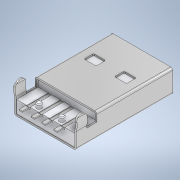
# Autodesk Inventor part: USB
Saved by Autodesk Inventor 2020 (Build 240168000, 168)
## iProperties
Created: 2022-06-10
Part Number: USB
Material: Типовые
Document SubType Name: Modeling
Designer: NoName
Density: 1 g/cm^3
Appearance: По умолчанию
Author: NoName
Autodesk Inventor part; units mm, degrees
ref_plane "YZ Plane" through (0, 0, 0) normal (1, 0, 0) x (0, 1, 0)
ref_plane "XZ Plane" through (0, 0, 0) normal (0, 1, 0) x (-1, 0, 0)
ref_plane "XY Plane" through (0, 0, 0) normal (0, 0, 1) x (1, 0, 0)
sketch "Эскиз1" plane through (0, 0, 0) normal (0, 0, 1) x (1, 0, 0)
  line L0 (-6, -2.25) -> (6, -2.25)
  line L1 (6, -2.25) -> (6, 2.25)
  line L2 (6, 2.25) -> (-6, 2.25)
  line L3 (-6, 2.25) -> (-6, -2.25)
  line L4 (-6, -2.25) -> (6, 2.25) construction
  line L5 (6, -2.25) -> (-6, 2.25) construction
  point P0 (0, 0)
  dimension "d0" = 12
  dimension "d1" = 4.5
  constraints: 12 end point, 2 midpoint, 2 parallel, 1 horizontal, 1 perpendicular
  measures "d0" distance between parallel lines of L1 L3
  measures "d1" distance between parallel lines of L0 L2
extrude "Выдавливание1" add sketch "Эскиз1" along normal blind 18.75
fillet "Сопряжение1" radius 0.4 4 edges at (6, 2.25, 9.375) (6, -2.25, 9.375) (-6, 2.25, 9.375) (-6, -2.25, 9.375)
shell "Оболочка1" thickness 0.3 removed faces 2 at (1.8667, -0.75, 18.75) at (1.8667, -0.75, 0)
sketch "Эскиз7" plane through (-5.6, -2.25, 0) normal (0, -1, 0) x (1, 0, 0)
  line L0 (1.675, 5.25) -> (3.6, 5.25)
  line L1 (3.8, 5.45) -> (3.8, 6.9)
  line L2 (3.6, 7.1) -> (1.675, 7.1)
  line L3 (1.475, 6.9) -> (1.475, 5.45)
  line L4 (7.6, 5.25) -> (9.525, 5.25)
  line L5 (9.725, 5.45) -> (9.725, 6.9)
  line L6 (9.525, 7.1) -> (7.6, 7.1)
  line L7 (7.4, 6.9) -> (7.4, 5.45)
  line L8 (5.6, 0) -> (5.6, 18.75)
  line L9 (0, 18.75) -> (11.2, 18.75) projected
  line L10 (0, 0) -> (11.2, 0) projected
  arc A0 (1.675, 7.1) -> (1.475, 6.9) centre (1.675, 6.9) ccw
  arc A1 (3.8, 6.9) -> (3.6, 7.1) centre (3.6, 6.9) ccw
  arc A2 (3.6, 5.25) -> (3.8, 5.45) centre (3.6, 5.45) ccw
  arc A3 (1.475, 5.45) -> (1.675, 5.25) centre (1.675, 5.45) ccw
  arc A4 (7.4, 5.45) -> (7.6, 5.25) centre (7.6, 5.45) ccw
  arc A5 (7.6, 7.1) -> (7.4, 6.9) centre (7.6, 6.9) ccw
  arc A6 (9.725, 6.9) -> (9.525, 7.1) centre (9.525, 6.9) ccw
  arc A7 (9.525, 5.25) -> (9.725, 5.45) centre (9.525, 5.45) ccw
  point P0 (1.475, 5.25)
  point P1 (3.8, 7.1)
  point P2 (3.8, 5.25)
  point P3 (1.475, 7.1)
  point P4 (7.4, 5.25)
  point P5 (9.725, 7.1)
  point P6 (9.725, 5.25)
  point P7 (7.4, 7.1)
  dimension "d32" = 3.6
  dimension "d33" = 8.25
  dimension "d34" = 1.85
  dimension "d35" = 5.25
  dimension "d38" = 0.2
  constraints: 18 end point, 16 point on circle, 16 point on line, 16 tangent, 8 centre point, 7 equal radius, 4 parallel, 2 horizontal, 2 perpendicular, 1 midpoint, 4 other
  measures "d32" distance between parallel lines of L7 L1
  measures "d33" distance between parallel lines of L5 L3
  measures "d34" distance between parallel lines of L0 L2
  measures "d35" distance between parallel lines of L10 L0
  measures "d38" radius of A0
extrude "Выдавливание6" cut sketch "Эскиз7" against normal through all
sketch "Эскиз5" plane through (0, 0, 0) normal (1, 0, 0) x (0, 1, 0)
  line L0 (2.25, 0) -> (1.85, 0) projected
  line L1 (1.95, 0.1) -> (-0.05, 0.1)
  line L2 (-0.05, 0.1) -> (-0.05, 8.6)
  line L3 (-0.05, 8.6) -> (1.95, 8.6)
  line L4 (1.95, 8.6) -> (1.95, 0)
  line L5 (-1.95, 0) -> (-1.95, 18.75) projected
  line L6 (1.95, 8.6) -> (-1.95, 8.6)
  line L7 (-1.95, 8.6) -> (-1.95, 14.45)
  line L8 (-1.95, 14.45) -> (1.95, 14.45)
  line L9 (1.95, 14.45) -> (1.95, 8.6)
  line L10 (-1.95, 14.45) -> (0.45, 14.45)
  line L11 (0.45, 14.45) -> (0.45, 18.65)
  line L12 (0.45, 18.65) -> (-1.95, 18.65)
  line L13 (-1.95, 18.65) -> (-1.95, 14.45)
  line L14 (1.95, 18.75) -> (1.95, 0) projected
  line L15 (1.85, 0) -> (-1.85, 0) projected
  line L16 (-1.85, 18.75) -> (1.85, 18.75) projected
  line L17 (-2.25, 0) -> (-2.25, 18.75) projected
  point P0 (0, 0)
  dimension "d20" = 2
  dimension "d21" = 0.1
  dimension "d22" = 0.1
  dimension "d23" = 8.6
  dimension "d24" = 4.3
  dimension "d25" = 2.7
  constraints: 24 end point, 6 parallel, 4 point on line, 3 horizontal, 3 perpendicular
  measures "d20" distance between parallel lines of L4 L2
  measures "d21" distance between parallel lines of L15 L1
  measures "d22" distance between parallel lines of L16 L12
  measures "d23" distance between parallel lines of L15 L6
  measures "d24" distance between parallel lines of L16 L8
  measures "d25" distance between parallel lines of L17 L11
extrude "Выдавливание4" add sketch "Эскиз5" along normal mid plane 11.5
sketch "Эскиз6" plane through (-6, -1.85, 0) normal (-1, 0, 0) x (0, 0, 1)
  line L0 (14.75, 2.4) -> (18.75, 2.4)
  line L1 (18.75, 2.4) -> (18.75, 4.1)
  line L2 (18.75, 4.1) -> (14.75, 4.1)
  line L3 (14.75, 4.1) -> (14.75, 2.4)
  line L4 (0, -0.4) -> (18.75, -0.4) projected
  point P0 (0, 1.85)
  dimension "d28" = 2.8
  dimension "d29" = 4
  constraints: 8 end point, 2 parallel, 1 coincident, 1 horizontal, 1 perpendicular
  measures "d28" distance between parallel lines of L4 L0
  measures "d29" distance between parallel lines of L1 L3
extrude "Выдавливание5" cut sketch "Эскиз6" against normal through all
sketch "Эскиз8" plane through (-5.7, 0.45, 18.65) normal (0, 1, 0) x (1, 0, 0)
  circle A0 centre (7.9, 0.9) radius 0.5
  circle A1 centre (3.5, 0.9) radius 0.5
  line L0 (11.3, 3.9) -> (0.1, 3.9) projected
  line L1 (5.7, 3.9) -> (5.7, -0.1)
  line L2 (11.3, -0.1) -> (0.1, -0.1) projected
  point P0 (5.7, 18.65)
  dimension "d39" = 1
  dimension "d40" = 4.4
  dimension "d41" = 1
  constraints: 2 centre point, 2 end point, 2 midpoint, 1 equal radius, 1 other
  measures "d39" diameter of A0
  measures "d40" distance of A1.centre A0.centre
  measures "d41" distance from line of L2 A1.centre
extrude "Выдавливание7" add sketch "Эскиз8" along normal blind 0.8
chamfer "Фаска2" distance 0.15 angle 45 2 edges at (1.7, 1.25, 17.75) (-2.7, 1.25, 17.75)
sketch "Эскиз9" plane through (-5.7, 0.45, 18.65) normal (0, 1, 0) x (1, 0, 0)
  line L0 (11.4, 4.2) -> (0, 4.2) projected
  line L1 (0, 0) -> (11.4, 0) construction
  line L2 (9.4, 4.2) -> (8.75, 4.2)
  line L3 (8.75, 4.2) -> (8.75, 0)
  line L4 (8.75, 0) -> (9.4, 0)
  line L5 (9.4, 0) -> (9.4, 4.2)
  line L6 (7.05, 0) -> (6.4, 0)
  line L7 (6.4, 0) -> (6.4, 4.2)
  line L8 (6.4, 4.2) -> (7.05, 4.2)
  line L9 (7.05, 4.2) -> (7.05, 0)
  line L10 (11.7, 3.9) -> (11.7, -0.1) projected
  line L11 (5.7, 4.2) -> (5.7, 0)
  line L12 (2, 4.2) -> (2.65, 4.2)
  line L13 (2.65, 4.2) -> (2.65, 0)
  line L14 (2.65, 0) -> (2, 0)
  line L15 (2, 0) -> (2, 4.2)
  line L16 (4.35, 0) -> (5, 0)
  line L17 (5, 0) -> (5, 4.2)
  line L18 (5, 4.2) -> (4.35, 4.2)
  line L19 (4.35, 4.2) -> (4.35, 0)
  point P0 (5.7, 18.65)
  dimension "d47" = 0.65
  dimension "d48" = 0.65
  dimension "d49" = 4.65
  dimension "d50" = 2.3
  constraints: 34 end point, 8 symmetric about line, 6 point on line, 4 parallel, 2 horizontal, 2 midpoint, 2 perpendicular
  measures "d47" distance between parallel lines of L7 L9
  measures "d48" distance between parallel lines of L5 L3
  measures "d49" distance between parallel lines of L10 L9
  measures "d50" distance between parallel lines of L10 L5
extrude "Выдавливание8" cut sketch "Эскиз9" against normal blind 0.1
sketch "Эскиз10" plane through (3.05, 0.45, 18.65) normal (1, 0, 0) x (0, 0, -1)
  line L0 (0, 0) -> (4.2, 0) projected
  line L1 (0, -0.1) -> (4.2, -0.1) projected
  line L2 (4.2, 0) -> (4.2, -0.1) projected
  line L3 (0, -0.1) -> (-0.1414, 0.0414)
  line L4 (-0.2828, 0.1) -> (-1.5, 0.1)
  line L5 (0, -2.3) -> (0, 0) projected
  line L6 (-1.5, 0.1) -> (-1.5, -0.1)
  line L7 (-1.5, -0.1) -> (-0.3657, -0.1)
  line L8 (-0.2243, -0.1586) -> (0, -0.3828)
  line L9 (-0.1, -2.3) -> (-0.1, 0.1) projected
  arc A0 (-0.1414, 0.0414) -> (-0.2828, 0.1) centre (-0.2828, -0.1) ccw
  arc A1 (-0.2243, -0.1586) -> (-0.3657, -0.1) centre (-0.3657, -0.3) ccw
  line L10 (0, -0.1) -> (0, 0) projected
  point P0 (18.65, -0.45)
  point P1 (-0.2828, -0.1)
  dimension "d54" = 0.2
  dimension "d55" = 0.2
  dimension "d56" = 1.4
  dimension "d57" = 0.2
  constraints: 10 end point, 4 point on circle, 4 tangent, 3 perpendicular, 3 point on line, 2 centre point, 1 equal radius, 1 horizontal alignment, 1 parallel
  measures "d54" distance between parallel lines of L4 L7
  measures "d55" distance between parallel lines of L3 L8
  measures "d56" distance between parallel lines of L9 L6
  measures "d57" radius of A0
extrude "Выдавливание9" add sketch "Эскиз10" along normal up to surface (0.65 mm away) contours L5 L8 L9 L3 | L9 L8 A1 L7 L6 L4 A0 L3
chamfer "Фаска3" distance 0.6 angle 45 1 edges at (0, -0.05, 0.1)
sketch "Эскиз11" plane through (-5.7, -0.05, 8.6) normal (0, -1, 0) x (1, 0, 0)
  line L0 (11.4, -7.9) -> (0, -7.9) projected
  line L1 (11.4, 0) -> (11.4, -7.9) projected
  line L2 (0, 0) -> (11.4, 0) projected
  line L3 (0, -7.9) -> (0, 0) projected
  line L4 (8.75, 10.05) -> (8.75, 5.85) projected
  line L5 (9.4, 5.85) -> (9.4, 10.05) projected
  line L6 (8.75, 5.85) -> (9.4, 5.85) projected
  line L7 (7.05, 5.85) -> (7.05, 10.05) projected
  line L8 (6.4, 5.85) -> (7.05, 5.85) projected
  line L9 (6.4, 10.05) -> (6.4, 5.85) projected
  line L10 (5, 5.85) -> (5, 10.05) projected
  line L11 (4.35, 5.85) -> (5, 5.85) projected
  line L12 (4.35, 10.05) -> (4.35, 5.85) projected
  line L13 (2.65, 5.85) -> (2.65, 10.05) projected
  line L14 (2, 5.85) -> (2.65, 5.85) projected
  line L15 (2, 10.05) -> (2, 5.85) projected
  line L16 (0.1, 0) -> (11.3, 0) projected
  line L17 (9.675, 0) -> (8.475, 0)
  line L18 (8.475, 0) -> (8.475, -7.6)
  line L19 (8.475, -7.6) -> (9.675, -7.6)
  line L20 (9.675, -7.6) -> (9.675, 0)
  line L21 (0.1, -8.6) -> (11.3, -8.6) projected
  line L22 (7.325, 0) -> (6.125, 0)
  line L23 (6.125, 0) -> (6.125, -6.1)
  line L24 (6.125, -6.1) -> (7.325, -6.1)
  line L25 (7.325, -6.1) -> (7.325, 0)
  line L26 (5.7, -8.6) -> (5.7, 0)
  line L27 (1.725, 0) -> (2.925, 0)
  line L28 (2.925, 0) -> (2.925, -7.6)
  line L29 (2.925, -7.6) -> (1.725, -7.6)
  line L30 (1.725, -7.6) -> (1.725, 0)
  line L31 (4.075, 0) -> (5.275, 0)
  line L32 (5.275, 0) -> (5.275, -6.1)
  line L33 (5.275, -6.1) -> (4.075, -6.1)
  line L34 (4.075, -6.1) -> (4.075, 0)
  line L35 (2.65, 10.05) -> (2, 10.05) projected
  line L36 (5, 10.05) -> (4.35, 10.05) projected
  line L37 (7.05, 10.05) -> (6.4, 10.05) projected
  line L38 (9.4, 10.05) -> (8.75, 10.05) projected
  point P0 (9.075, 0)
  point P1 (9.075, 5.85)
  point P2 (6.725, 0)
  point P3 (6.725, 5.85)
  point P4 (2.325, 0)
  point P5 (4.675, 0)
  point P6 (9.675, 0)
  point P7 (8.475, 0)
  point P8 (2.925, 0)
  point P9 (1.725, 0)
  dimension "d63" = 1.2
  dimension "d64" = 1
  dimension "d65" = 2.5
  constraints: 34 end point, 10 symmetric about line, 5 midpoint, 5 parallel, 2 horizontal, 2 perpendicular, 2 point on line, 2 vertical alignment
  measures "d63" distance between parallel lines of L18 L20
  measures "d64" distance between parallel lines of L21 L19
  measures "d65" distance between parallel lines of L21 L24
extrude "Выдавливание10" cut sketch "Эскиз11" against normal blind 0.1 contours L32 L33 L34 L2 | L2 L25 L24 L23 | L20 L19 L18 L2 | L2 L28 L29 L30
pattern_linear "Прямоуг.массив1" count 2 spacing 2.35 along (-1, 0, 0) of "Выдавливание9"
mirror "Зеркальное отражение1" about plane through (0, 0, 0) normal (1, 0, 0) of "Выдавливание9", "Прямоуг.массив1"
sketch "Эскиз12" plane through (0, 0, 18.75) normal (0, 0, 1) x (1, 0, 0)
  line L0 (6, 1.85) -> (6, 0.55) projected
  line L1 (6, 0.55) -> (5.7, 0.55)
  line L2 (5.7, 0.55) -> (5.7, 3.45) construction
  line L3 (5.7, 3.45) -> (6, 3.45)
  line L4 (6, 3.45) -> (6, 0.55) construction
  line L5 (-5.6, -2.25) -> (5.6, -2.25) projected
  arc A0 (6, 0.944) -> (6, 3.056) centre (3.192, 2) ccw
  line L6 (5.7, 0.55) -> (5.7, 1.85) projected
  arc A1 (5.7, 1) -> (5.7, 3) centre (3.192, 2) ccw
  line L7 (5.7, 3) -> (5.7, 3.45)
  line L8 (6, 3.45) -> (6, 3.056)
  line L9 (6, 0.944) -> (6, 0.55)
  line L10 (6, -1.85) -> (6, 1.85) projected
  line L11 (5.7, 1) -> (5.7, 0.55)
  line L12 (5.7, -1.85) -> (5.7, 1.85) projected
  point P0 (0, 0)
  point P1 (6, 0.944)
  dimension "d84" = 5.7
  dimension "d85" = 0.3
  dimension "d86" = 3
  dimension "d87" = 2
  dimension "d88" = 4.25
  constraints: 16 end point, 5 point on line, 4 point on circle, 3 collinear, 2 centre point, 2 parallel, 1 coincident, 1 horizontal, 1 perpendicular, 1 vertical
  measures "d84" distance between parallel lines of L3 L5
  measures "d85" radial gap between concentric circles of A0 A1
  measures "d86" radius of A0
  measures "d87" distance of L11.start L7.start
  measures "d88" distance from line of L5 A0.centre
extrude "Выдавливание11" add sketch "Эскиз12" against normal blind 2
sketch "Эскиз14" plane through (5.7, 3, 18.75) normal (-1, 0, 0) x (0, 0, 1)
  line L0 (-2, -2) -> (-2, 0) projected
  arc A0 (0, -0.55) -> (-2, -0.55) centre (-1, -0.55) ccw
  line L1 (0, 0) -> (0, -2) projected
  line L2 (0, 0.45) -> (-2, 0.45) projected
  line L3 (-2, 0.45) -> (-2, 0.056) projected
  line L4 (-2, -0.55) -> (-2, 0.45)
  line L5 (0, 0.056) -> (0, 0.45) projected
  line L6 (-2, 0.45) -> (0, 0.45)
  line L7 (0, 0.45) -> (0, -0.55)
  line L8 (0, -2.056) -> (0, 0.056) projected
  point P0 (-18.75, -3)
  point P1 (-1, 0.45)
  point P2 (0, -0.55)
  dimension "d89" = 1
  constraints: 6 end point, 3 tangent, 2 horizontal alignment, 2 point on circle, 1 centre point, 1 collinear, 1 perpendicular, 1 point on line, 1 vertical
  measures "d89" distance from line of L2 A0.centre
extrude "Выдавливание13" cut sketch "Эскиз14" against normal through all
mirror "Зеркальное отражение3" about plane through (0, 0, 0) normal (1, 0, 0) of "Выдавливание13", "Выдавливание11"
